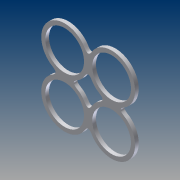
# Autodesk Inventor part: PropProtector
Saved by Autodesk Inventor 2011 SP1 (Build 150282100, 282)
## iProperties
Created: 2011-08-22
Part Number: PropProtector
Document SubType Name: Modeling
Designer: Nathan
Density: 1 g/cm^3
Author: Nathan
Autodesk Inventor part; units mm, degrees
ref_plane "YZ Plane" through (0, 0, 0) normal (1, 0, 0) x (0, 1, 0)
ref_plane "XZ Plane" through (0, 0, 0) normal (0, 1, 0) x (-1, 0, 0)
ref_plane "XY Plane" through (0, 0, 0) normal (0, 0, 1) x (1, 0, 0)
sketch "Sketch1" plane through (0, 0, 0) normal (0, 0, 1) x (1, 0, 0)
  line L0 (0, 0) -> (71.842, 71.842)
  line L1 (0, 0) -> (101.6, 0) construction
  line L2 (0, 0) -> (-71.842, 71.842)
  line L3 (0, 0) -> (101.6, 0) construction
  circle A0 centre (-161.6446, 161.6446) radius 133.35
  line L4 (0, 0) -> (101.6, 0)
  arc A1 (-39.7375, 267.2529) -> (-267.2529, 39.7375) centre (-161.6446, 161.6446) ccw
  circle A2 centre (161.6446, -161.6446) radius 133.35
  arc A3 (39.7375, -267.2529) -> (267.2529, -39.7375) centre (161.6446, -161.6446) ccw
  circle A4 centre (-161.6446, -161.6446) radius 133.35
  arc A5 (-267.2529, -39.7375) -> (-39.7375, -267.2529) centre (-161.6446, -161.6446) ccw
  arc A6 (267.2529, 39.7375) -> (39.7375, 267.2529) centre (161.6446, 161.6446) ccw
  circle A7 centre (161.6446, 161.6446) radius 133.35
  spline S0 degree 4 poles (-39.7375, 267.2529) (-20.5214, 245.0712) (0, 181.6818) (20.5214, 245.0712) (39.7375, 267.2529) knots 0 0 0 0 0 1 1 1 1 1
  spline S1 degree 4 poles (-39.7375, -267.2529) (-20.5214, -245.0712) (0, -181.6818) (20.5214, -245.0712) (39.7375, -267.2529) knots 0 0 0 0 0 1 1 1 1 1
  spline S2 degree 4 poles (-267.2529, 39.7375) (-245.0712, 20.5214) (-181.6818, 0) (-245.0712, -20.5214) (-267.2529, -39.7375) knots 0 0 0 0 0 1 1 1 1 1
  spline S3 degree 4 poles (267.2529, 39.7375) (245.0712, 20.5214) (181.6818, 0) (245.0712, -20.5214) (267.2529, -39.7375) knots 0 0 0 0 0 1 1 1 1 1
  line L5 (-161.6446, 161.6446) -> (-161.6446, 89.6025)
  line L6 (-161.6446, 161.6446) -> (-76.5569, 161.6446)
  line L7 (161.6446, -161.6446) -> (161.6446, -113.6338)
  line L8 (161.6446, -161.6446) -> (107.4543, -161.6446)
  arc A8 (56.0363, -39.7375) -> (39.7375, -56.0363) centre (161.6446, -161.6446) ccw
  arc A9 (39.7375, 56.0363) -> (56.0363, 39.7375) centre (161.6446, 161.6446) ccw
  arc A10 (-56.0363, 39.7375) -> (-39.7375, 56.0363) centre (-161.6446, 161.6446) ccw
  arc A11 (-39.7375, -56.0363) -> (-56.0363, -39.7375) centre (-157.2611, -157.2611) ccw
  spline S4 degree 4 poles (-56.0363, 39.7375) (-78.218, 20.5214) (-141.5702, 0.0417) (-78.2738, -20.584) (-56.0363, -39.7375) knots 0 0 0 0 0 1 1 1 1 1
  spline S5 degree 4 poles (-39.7375, -56.0363) (-20.584, -78.2738) (0.0417, -141.5702) (20.5214, -78.218) (39.7375, -56.0363) knots 0 0 0 0 0 1 1 1 1 1
  spline S6 degree 4 poles (-39.7375, 56.0363) (-20.5214, 78.218) (0, 141.6074) (20.5214, 78.218) (39.7375, 56.0363) knots 0 0 0 0 0 1 1 1 1 1
  spline S7 degree 4 poles (56.0363, 39.7375) (78.218, 20.5214) (141.6074, 0) (78.218, -20.5214) (56.0363, -39.7375) knots 0 0 0 0 0 1 1 1 1 1
  point P0 (0, 224.0729)
  point P1 (0, -224.0729)
  point P2 (-224.0729, 0)
  point P3 (224.0729, 0)
  point P4 (-99.2163, 0)
  point P5 (0, -99.2163)
  point P6 (0, 99.2163)
  point P7 (99.2163, 0)
  dimension "d0" = 101.6
  dimension "d1" = 45
  dimension "d2" = 101.6
  dimension "d3" = 135
  dimension "d5" = 228.6
  dimension "d7" = 266.7
  dimension "d9" = 0
  dimension "d14" = 27.94
  dimension "d15" = 0
  dimension "d17" = 0
  dimension "d26" = 43.18
  constraints: 27 symmetric about line, 18 end point, 17 point on circle, 12 centre point, 7 coincident, 5 perpendicular, 2 equal length, 2 horizontal, 1 collinear, 1 point on line, 48 other
  measures "d0" distance of L0.start L0.end
  measures "d1" angle of L1 L0
  measures "d2" distance of L0.start L2.end
  measures "d3" angle of L3 L2
  measures "d5" distance from line of L0 A0.centre
  measures "d7" diameter of A0
  measures "d9" vertical distance of A6.end point (-39.737, 267.253)
  measures "d14" radial gap between concentric circles of A1 A0
  measures "d15" horizontal distance of A5.start A1.end
  measures "d17" horizontal distance of A6.start A3.end
  measures "d26" vertical distance of A3.start point (0, -224.073)
extrude "Extrusion3" add sketch "Sketch1" along normal blind 25.4
body "Solid3"
